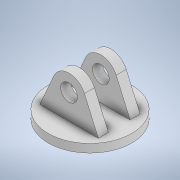
# Autodesk Inventor part: New_Arm_plate
Saved by Autodesk Inventor 2021 (Build 250183000, 183)
## iProperties
Created: 2021-08-05
Part Number: New_Arm_plate
Material: Generic
Document SubType Name: Modeling
Designer: hp
Density: 1 g/cm^3
Appearance: Default
Author: hp
Autodesk Inventor part; units mm, degrees
ref_plane "YZ Plane" through (0, 0, 0) normal (1, 0, 0) x (0, 1, 0)
ref_plane "XZ Plane" through (0, 0, 0) normal (0, 1, 0) x (-1, 0, 0)
sketch "Sketch1" plane through (0, 0, 0) normal (0, 1, 0) x (-1, 0, 0)
  circle A0 centre (0, 0) radius 5
  dimension "d0" = 10
  constraints: 1 centre point, 1 coincident
  measures "d0" diameter of A0
extrude "Extrusion1" add sketch "Sketch1" along normal blind 1
ref_plane "Work Plane1" through (0, 0, 0) normal (0, 0, 1) x (1, 0, 0)
sketch "Sketch2" plane through (0, 0, 0) normal (0, 0, 1) x (1, 0, 0)
  line L0 (0, 0) -> (0, 4)
  circle A0 centre (0, 4) radius 1
  circle A1 centre (0, 4) radius 2
  line L1 (5, 1) -> (-5, 1) projected
  line L2 (0, 1) -> (3.5, 1)
  line L3 (0, 1) -> (-3.5, 1)
  line L4 (-3.5, 1) -> (-1.8315, 4.8034)
  line L5 (3.5, 1) -> (1.8315, 4.8034)
  dimension "d4" = 4
  dimension "d5" = 2
  dimension "d6" = 4
  dimension "d7" = 3.5
  dimension "d8" = 3.5
  constraints: 10 end point, 2 centre point, 2 coincident, 2 point on circle, 2 point on line, 2 tangent, 1 midpoint, 1 vertical
  measures "d4" distance of L0.start L0.end
  measures "d5" diameter of A0
  measures "d6" diameter of A1
  measures "d7" distance of L2.start L2.end
  measures "d8" distance of L2.start L3.end
extrude "Extrusion2" add sketch "Sketch2" along normal mid plane 5
sketch "Sketch3" plane through (0, 0, 0) normal (0, 0, 1) x (1, 0, 0)
  arc A0 (1.8315, 4.8034) -> (-1.8315, 4.8034) centre (0, 4) ccw projected
  circle A1 centre (0, 4) radius 1
  circle A2 centre (0, 4) radius 2
  line L0 (-1.8315, 4.8034) -> (-3.5, 1) projected
  line L1 (-1.8315, 4.8034) -> (-3.5, 1)
  line L2 (5, 1) -> (-5, 1) projected
  line L3 (3.5, 1) -> (1.8315, 4.8034) projected
  line L4 (1.8315, 4.8034) -> (3.5, 1)
  line L5 (3.5, 1) -> (-3.5, 1)
  point P0 (0, 0)
  dimension "d11" = 4
  constraints: 6 end point, 2 centre point, 2 coincident, 1 collinear, 1 horizontal, 1 point on line
  measures "d11" diameter of A2
extrude "Extrusion3" cut sketch "Sketch3" along normal mid plane 2.6 contours A2 A0 | L3 L2 L0 A2 | A1
body "Solid1"
